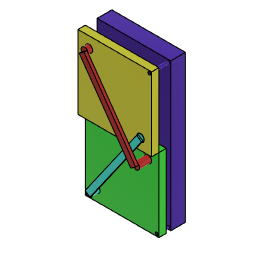
Evolution Door v6 (Autodesk Fusion 360 design; units mm, degrees)
Autodesk Fusion 360 part; units mm, degrees
note: some values were not read from the file. Set by a fixed rule: which face or edge a step refers to.
sketch "Wall" plane through (0, 0, 0) normal (0, 1, 0) x (1, 0, 0) in component "Wall"
  line L0 (0, 0) -> (-50, 0)
  line L1 (-50, 0) -> (-50, -100)
  line L2 (-50, -100) -> (0, -100)
  line L3 (0, -100) -> (0, 0)
  dimension "d1" = 50
  dimension "d2" = 100
  constraint horizontal L0
  constraint vertical L1
  constraint horizontal L2
  constraint vertical L3
  constraint coincident L0.start L3.end
  measures "d1" distance of L0.start L0.end
  measures "d2" distance of L0.start L2.end
extrude "Extrude1" add sketch "Wall" against normal blind 10 makes body 1 in component "Wall"
ref_plane "WorkPlane1" through (-25, -13, 50) normal (0, -1, 0) x (0, 0, -1) in component "Door Down"
sketch "Door Down" plane through (-25, -13, 50) normal (0, -1, 0) x (1, 0, 0) in component "Door Down"
  line L0 (25, -50) -> (-25, -50)
  line L1 (-25, -50) -> (-25, 0)
  line L2 (-25, 0) -> (25, 0)
  line L3 (25, 0) -> (25, -50)
  line L4 (0, 0) -> (0, -50) construction
  line L5 (-25, -25) -> (25, -25) construction
  circle A0 centre (17.5, -7.5) radius 2.5495
  circle A1 centre (-17.5, -42.5) radius 2.5495
  circle A2 centre (23.5, -48.5) radius 1
  constraint horizontal L0
  constraint vertical L1
  constraint horizontal L2
  constraint vertical L3
  constraint coincident L4.start origin
  constraint midpoint L0 L4.end
  constraint perpendicular L0 L4
  constraint midpoint L1 L5.start
  constraint midpoint L3 L5.end
extrude "Extrude1'" add sketch "Door Down" along normal blind 5 separate body contours L0 L1 L2 L3 | A0 | A1 makes body 2 in component "Door Down"
extrude "Extrude2" cut sketch "Door Down" along normal blind 8 contours A0 bodies 2 in component "Door Down"
extrude "Extrude3" cut sketch "Door Down" along normal blind 6 contours A1 bodies 2 in component "Door Down"
extrude "Extrude2'" add sketch "Door Down" along normal blind 5 and the other way blind 3 contours A2 bodies 1 in component "Wall"
sketch "Door Up" plane through (0, -18, 0) normal (0, -1, 0) x (1, 0, 0) in component "Door Up"
  circle A0 centre (-42.5, 7.5) radius 2.5495
  circle A1 centre (-7.5, 42.5) radius 2.5495
  circle A2 centre (-1.5, 1.5) radius 1
  line L0 (0, 50) -> (-50, 50)
  line L1 (-50, 50) -> (-50, 0)
  line L2 (-50, 0) -> (0, 0)
  line L3 (0, 0) -> (0, 50)
  line L4 (-50, 100) -> (0, 100)
  line L5 (0, 100) -> (0, 50)
  line L6 (0, 50) -> (-50, 50)
  line L7 (-50, 50) -> (-50, 100)
  line L8 (-50, 50) -> (0, 50) construction
  circle A3 centre (-7.5, 57.5) radius 2.5495
  circle A4 centre (-42.5, 92.5) radius 2.5495
  circle A5 centre (-1.5, 98.5) radius 1
  constraint horizontal L4
  constraint vertical L5
  constraint horizontal L6
  constraint vertical L7
  constraint coincident L0.start L3.end
extrude "Extrude1''" add sketch "Door Up" along normal blind 5 separate body contours L0 L4 L5 L6 L7 makes body 3 in component "Door Up"
extrude "Extrude3'" add sketch "Door Up" along normal blind -8 and the other way blind -5 contours A5 bodies 1 in component "Wall"
move_face "OffsetFaces1" offset -0.1 1 faces at (-0.5012, -12.6667, 1.4502) on bodies 1 in component "Wall"
move_face "OffsetFaces2" offset -0.1 1 faces at (-0.5012, -18.6667, 98.5498) on bodies 1 in component "Wall"
sketch "Left Down Link" plane through (0, -23, 0) normal (0, -1, 0) x (1, 0, 0) in component "Left Down Link"
  circle A0 centre (-1.5, 98.5) radius 1
  circle A1 centre (-42.5, 92.5) radius 2.5495
  circle A2 centre (-7.5, 57.5) radius 2.5495
  line L0 (-50, 50) -> (0, 50)
  line L1 (0, 50) -> (0, 100)
  line L2 (0, 100) -> (-50, 100)
  line L3 (-50, 100) -> (-50, 50)
  circle A3 centre (-7.5, 57.5) radius 2.5495
  circle A4 centre (-42.4941, 7.505) radius 2.5495
  line L4 (-7.5, 57.5) -> (-42.4941, 7.505)
  line L5 (-42.4941, 7.505) -> (-40.8556, 6.3582)
  line L6 (-40.8556, 6.3582) -> (-5.8616, 56.3529)
  line L7 (-5.8616, 56.3529) -> (-7.5, 57.5)
  line L8 (-44.1326, 8.6519) -> (-9.1386, 58.6467)
  line L9 (-9.1386, 58.6467) -> (-7.5, 57.5)
  line L10 (-42.4941, 7.505) -> (-44.1326, 8.6519)
  dimension "d32" = 5.099
  dimension "d33" = 2
  dimension "d34" = 61.025
  constraint concentric A2 A3
  constraint coincident A2.centre A3.centre
  constraint coincident A4.centre L4.end
  constraint perpendicular L4 L5
  constraint perpendicular L5 L6
  constraint symmetric A4.centre L4 L5.start
  constraint symmetric L4 L5.end L8.start
  constraint symmetric L4 L6.end L8.end
  constraint symmetric L4 A2.centre A3.centre
  measures "d32" diameter of A4
  measures "d33" distance of A4.centre L5.end
  measures "d34" distance of L5.end L6.end
extrude "Extrude1'''" add sketch "Left Down Link" against normal blind 5 separate body contours A2 A3 L6 L7 L8 L9 | A2 A3 L4 L8 L9 | A2 A3 L4 L6 L7 makes body 4 in component "Left Down Link"
extrude "Extrude2''" add sketch "Left Down Link" against normal blind 10 separate body contours A4 L5 L6 L8 L10 | A4 L4 L8 L10 | A4 L4 L5 L6 makes body 5 in component "Left Down Link"
move_face "OffsetFaces1'" offset -0.2 1 faces at (-41.5107, -16.3333, 9.8573) on bodies 5 in component "Left Down Link"
move_face "OffsetFaces2'" offset -0.2 1 faces at (-6.8737, -19.6667, 55.0286) on bodies 4 in component "Left Down Link"
extrude "Extrude3''" add sketch "Left Down Link" along normal blind 1 contours A2 A3 L4 L8 L9 | A2 L0 A3 L4 L8 | A2 L0 A3 L4 L6 | A2 A3 L4 L6 L7 | L0 A4 L4 L8 | L0 A4 L4 L6 | A4 L4 L8 L10 | A4 L4 L5 L6 bodies 4 5 in component "Left Down Link"
ref_plane "WorkPlane1" through (-25, -26, 75) normal (0, -1, 0) x (1, 0, 0) in component "Left Up Link"
sketch "Left Up Link" plane through (-25, -26, 75) normal (0, -1, 0) x (1, 0, 0) in component "Left Up Link"
  circle A0 centre (-17.5, 17.5) radius 2.5495
  circle A1 centre (17.5, -32.5) radius 2.5495
  line L0 (-17.5, 17.5) -> (17.5, -32.5)
  line L1 (17.5, -32.5) -> (19.1385, -31.3531)
  line L2 (-17.5, 17.5) -> (-15.8615, 18.6469)
  line L3 (-15.8615, 18.6469) -> (19.1385, -31.3531)
  line L4 (-19.1385, 16.3531) -> (15.8615, -33.6469)
  line L5 (-17.5, 17.5) -> (-19.1385, 16.3531)
  line L6 (17.5, -32.5) -> (15.8615, -33.6469)
  dimension "d44" = 5.099
  dimension "d45" = 2
  dimension "d46" = 2
  constraint coincident A0.centre L0.start
  constraint coincident A1.centre L0.end
  constraint perpendicular L0 L1
  constraint perpendicular L0 L2
  constraint perpendicular L1 L3
  constraint symmetric A1.centre L0 L1.start
  constraint symmetric L0 L1.end L4.end
  constraint symmetric L0 A0.centre L2.start
  constraint symmetric L0 L2.end L4.start
  measures "d44" diameter of A1
  measures "d45" distance of A1.centre L1.end
  measures "d46" distance of A0.centre L2.end
extrude "Extrude1''''" add sketch "Left Up Link" against normal blind 8 separate body contours A0 L2 L3 L4 L5 | A0 L0 L4 L5 | A0 L0 L2 L3 makes body 6 in component "Left Up Link"
extrude "Extrude2'''" add sketch "Left Up Link" against normal blind 13 separate body contours A1 L1 L3 L4 L6 | A1 L0 L4 L6 | A1 L0 L1 L3 makes body 7 in component "Left Up Link"
move_face "OffsetFaces1''" offset -0.2 1 faces at (-5.4915, -17.3333, 44.0703) on bodies 7 in component "Left Up Link"
move_face "OffsetFaces2''" offset -0.2 1 faces at (-39.9505, -20.6667, 92.4835) on bodies 6 in component "Left Up Link"
extrude "Extrude3'''" add sketch "Left Up Link" along normal blind 2 contours A0 L0 L4 L5 | A0 A1 L0 L4 | A0 A1 L0 L3 | A0 L0 L2 L3 | A1 L0 L4 L6 | A1 L0 L1 L3 bodies 6 7 in component "Left Up Link"
component "Wall" placed x (1, 0, 0) y (0, 1, 0) z (0, 0, 1) at (0, 0, 0)
component "Door Down" placed x (1, 0, 0) y (0, 1, 0) z (0, 0, 1) at (0, 0, 0)
component "Door Up" placed x (1, 0, 0) y (0, 1, 0) z (0, 0, 1) at (0, 0, 0)
component "Left Down Link" placed x (1, 0, 0) y (0, 1, 0) z (0, 0, 1) at (0, 0, 0)
component "Left Up Link" placed x (1, 0, 0) y (0, 1, 0) z (0, 0, 1) at (0, 0, 0)
named bodies: "Wall", "Door Down", "Left Down Link", "Left Up Link"
